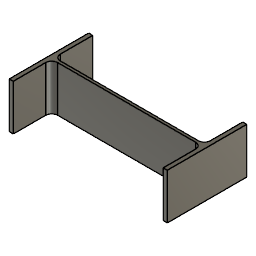
H-346×174×6×9 (Autodesk Fusion 360 design; units mm, degrees)
Autodesk Fusion 360 part; units mm, degrees
sketch "スケッチ1" plane through (0, 0, 0) normal (0, 0, 1) x (1, 0, 0)
  line L0 (0, 87) -> (0, -87)
  line L1 (346, -87) -> (346, 87)
  line L2 (337, -16) -> (337, -87)
  line L3 (9, -87) -> (9, -16)
  line L4 (0, -87) -> (9, -87)
  line L5 (337, -87) -> (346, -87)
  line L6 (9, 16) -> (9, 87)
  line L7 (337, 87) -> (337, 16)
  line L8 (324, 3) -> (22, 3)
  line L9 (22, -3) -> (324, -3)
  line L10 (9, 87) -> (0, 87)
  line L11 (346, 87) -> (337, 87)
  arc A0 (22, -3) -> (9, -16) centre (22, -16) ccw
  arc A1 (9, 16) -> (22, 3) centre (22, 16) ccw
  arc A2 (324, 3) -> (337, 16) centre (324, 16) ccw
  arc A3 (337, -16) -> (324, -3) centre (324, -16) ccw
extrude "押し出し1" add sketch "スケッチ1" along normal blind 100
